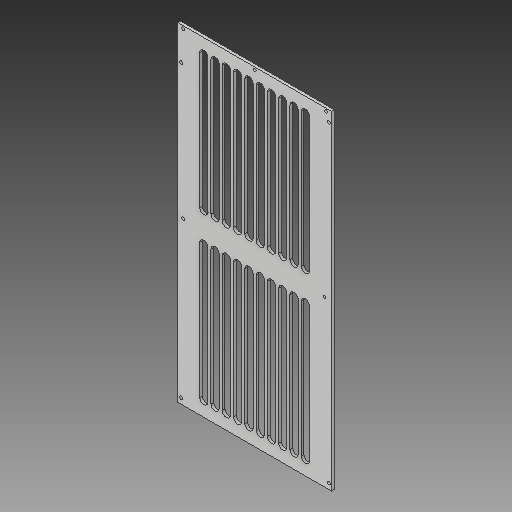
# Autodesk Inventor part: GlyphPlateUnderside
Saved by Autodesk Inventor 2019 (Build 230136000, 136)
## iProperties
Created: 2018-01-27
Part Number: GlyphPlateUnderside
Material: Generic
Document SubType Name: Modeling
Designer: User
Density: 1 g/cm^3
Appearance: Default
Author: User
Autodesk Inventor part; units mm, degrees
ref_plane "YZ Plane" through (0, 0, 0) normal (1, 0, 0) x (0, 1, 0)
ref_plane "XZ Plane" through (0, 0, 0) normal (0, 1, 0) x (-1, 0, 0)
ref_plane "XY Plane" through (0, 0, 0) normal (0, 0, 1) x (1, 0, 0)
sketch "Sketch1" plane through (0, 0, 0) normal (0, 0, 1) x (1, 0, 0)
  line L0 (0, 0) -> (178.2064, 0)
  line L1 (178.2064, 0) -> (178.2064, 381)
  line L2 (178.2064, 381) -> (0, 381)
  line L3 (0, 381) -> (0, 0)
  dimension "d0" = 178.2064
  dimension "d1" = 381
  constraints: 8 end point, 2 parallel, 1 horizontal, 1 perpendicular
  measures "d0" distance of L2.end L1.end
  measures "d1" distance of L1.end L0.end
extrude "Extrusion1" add sketch "Sketch1" along normal blind 3.175
sketch "Sketch2" plane through (0, 0, 3.175) normal (0, 0, 1) x (1, 0, 0)
  line L0 (0, 0) -> (178.2064, 0) projected
  line L1 (0, 0) -> (4.0386, 0)
  line L2 (4.0386, 0) -> (4.0386, 6.35)
  line L3 (0, 381) -> (0, 0) projected
  line L4 (0, 381) -> (4.0386, 381)
  line L5 (178.2064, 381) -> (0, 381) projected
  line L6 (4.0386, 381) -> (4.0386, 342.9)
  line L7 (4.0386, 381) -> (42.1386, 381) construction
  line L8 (0, 381) -> (0, 377.825)
  line L9 (0, 377.825) -> (6.35, 377.825)
  line L10 (178.2064, 0) -> (178.2064, 381) projected
  line L11 (178.2064, 0) -> (175.0314, 0)
  line L12 (175.0314, 0) -> (175.0314, 6.35)
  line L13 (178.2064, 377.825) -> (171.8564, 377.825)
  point P0 (175.0314, 368.3)
  dimension "d4" = 4.0386
  dimension "d5" = 6.35
  dimension "d6" = 38.1
  dimension "d7" = 90
  dimension "d8" = 3.175
  dimension "d9" = 6.35
  dimension "d10" = 3.175
  dimension "d11" = 6.35
  dimension "d19" = 4.0386
  dimension "d21" = 3.175
  dimension "d22" = 12.7
  dimension "d23" = 3.175
  constraints: 20 end point, 5 coincident, 5 perpendicular, 5 point on line, 1 horizontal, 1 vertical
  measures "d4" distance of L0.start L1.end
  measures "d5" distance of L1.end L2.end
  measures "d6" distance of L4.end L6.end
  measures "d7" angle of L6 L7
  measures "d8" distance of L3.start L8.end
  measures "d9" distance of L8.end L9.end
  measures "d10" distance of L0.end L11.end
  measures "d11" distance of L13.start L13.end
  measures "d19" distance between parallel lines of L3 L6
  measures "d21" distance from line of L10 point (175.031, 368.3)
  measures "d22" distance from line of point (175.031, 368.3) L5
  measures "d23" distance from line of L5 L13.end
hole "Hole1" at (4.0386, 6.35, 3.175) at (4.0386, 342.9, 3.175) at (6.35, 377.825, 3.175) at (175.0314, 6.35, 3.175) at (175.0314, 368.3, 3.175) at (171.8564, 377.825, 3.175) direction (0, 0, -1) diameter 3.556 depth 25.4 tip angle 118
sketch "Sketch3" plane through (0, 0, 3.175) normal (0, 0, 1) x (1, 0, 0)
  line L0 (30.1625, 12.7) -> (30.1625, 177.8) construction
  line L1 (34.925, 17.4625) -> (34.925, 173.0375)
  line L2 (25.4, 173.0375) -> (25.4, 17.4625)
  arc A0 (25.4, 17.4625) -> (34.925, 17.4625) centre (30.1625, 17.4625) ccw
  arc A1 (34.925, 173.0375) -> (25.4, 173.0375) centre (30.1625, 173.0375) ccw
  line L3 (0, 381) -> (0, 0) projected
  line L4 (178.2064, 0) -> (178.2064, 381) projected
  line L5 (0, 0) -> (178.2064, 0) projected
  line L6 (43.2435, 12.7) -> (43.2435, 177.8) construction
  line L7 (48.006, 17.4625) -> (48.006, 173.0375)
  line L8 (38.481, 173.0375) -> (38.481, 17.4625)
  arc A2 (38.481, 17.4625) -> (48.006, 17.4625) centre (43.2435, 17.4625) ccw
  arc A3 (48.006, 173.0375) -> (38.481, 173.0375) centre (43.2435, 173.0375) ccw
  line L9 (56.3245, 12.7) -> (56.3245, 177.8) construction
  line L10 (61.087, 17.4625) -> (61.087, 173.0375)
  line L11 (51.562, 173.0375) -> (51.562, 17.4625)
  arc A4 (51.562, 17.4625) -> (61.087, 17.4625) centre (56.3245, 17.4625) ccw
  arc A5 (61.087, 173.0375) -> (51.562, 173.0375) centre (56.3245, 173.0375) ccw
  line L12 (69.4055, 12.7) -> (69.4055, 177.8) construction
  line L13 (74.168, 17.4625) -> (74.168, 173.0375)
  line L14 (64.643, 173.0375) -> (64.643, 17.4625)
  arc A6 (64.643, 17.4625) -> (74.168, 17.4625) centre (69.4055, 17.4625) ccw
  arc A7 (74.168, 173.0375) -> (64.643, 173.0375) centre (69.4055, 173.0375) ccw
  line L15 (82.4865, 12.7) -> (82.4865, 177.8) construction
  line L16 (87.249, 17.4625) -> (87.249, 173.0375)
  line L17 (77.724, 173.0375) -> (77.724, 17.4625)
  arc A8 (77.724, 17.4625) -> (87.249, 17.4625) centre (82.4865, 17.4625) ccw
  arc A9 (87.249, 173.0375) -> (77.724, 173.0375) centre (82.4865, 173.0375) ccw
  line L18 (95.5675, 12.7) -> (95.5675, 177.8) construction
  line L19 (100.33, 17.4625) -> (100.33, 173.0375)
  line L20 (90.805, 173.0375) -> (90.805, 17.4625)
  arc A10 (90.805, 17.4625) -> (100.33, 17.4625) centre (95.5675, 17.4625) ccw
  arc A11 (100.33, 173.0375) -> (90.805, 173.0375) centre (95.5675, 173.0375) ccw
  line L21 (108.6485, 12.7) -> (108.6485, 177.8) construction
  line L22 (113.411, 17.4625) -> (113.411, 173.0375)
  line L23 (103.886, 173.0375) -> (103.886, 17.4625)
  arc A12 (103.886, 17.4625) -> (113.411, 17.4625) centre (108.6485, 17.4625) ccw
  arc A13 (113.411, 173.0375) -> (103.886, 173.0375) centre (108.6485, 173.0375) ccw
  line L24 (121.7295, 12.7) -> (121.7295, 177.8) construction
  line L25 (126.492, 17.4625) -> (126.492, 173.0375)
  line L26 (116.967, 173.0375) -> (116.967, 17.4625)
  arc A14 (116.967, 17.4625) -> (126.492, 17.4625) centre (121.7295, 17.4625) ccw
  arc A15 (126.492, 173.0375) -> (116.967, 173.0375) centre (121.7295, 173.0375) ccw
  line L27 (160.7328, 14.2764) -> (160.7328, 166.6986) construction
  line L28 (134.8105, 12.7) -> (134.8105, 177.8) construction
  line L29 (139.573, 17.4625) -> (139.573, 173.0375)
  line L30 (130.048, 173.0375) -> (130.048, 17.4625)
  arc A16 (130.048, 17.4625) -> (139.573, 17.4625) centre (134.8105, 17.4625) ccw
  arc A17 (139.573, 173.0375) -> (130.048, 173.0375) centre (134.8105, 173.0375) ccw
  line L31 (178.2064, 0) -> (178.2064, 381) projected
  line L32 (30.1625, 368.3) -> (30.1625, 203.2) construction
  line L33 (34.925, 363.5375) -> (34.925, 207.9625)
  line L34 (25.4, 207.9625) -> (25.4, 363.5375)
  arc A18 (34.925, 363.5375) -> (25.4, 363.5375) centre (30.1625, 363.5375) ccw
  arc A19 (25.4, 207.9625) -> (34.925, 207.9625) centre (30.1625, 207.9625) ccw
  arc A20 (38.481, 207.9625) -> (48.006, 207.9625) centre (43.2435, 207.9625) ccw
  line L35 (48.006, 363.5375) -> (48.006, 207.9625)
  line L36 (38.481, 207.9625) -> (38.481, 363.5375)
  line L37 (43.2435, 368.3) -> (43.2435, 203.2) construction
  arc A21 (48.006, 363.5375) -> (38.481, 363.5375) centre (43.2435, 363.5375) ccw
  arc A22 (51.562, 207.9625) -> (61.087, 207.9625) centre (56.3245, 207.9625) ccw
  line L38 (61.087, 363.5375) -> (61.087, 207.9625)
  line L39 (51.562, 207.9625) -> (51.562, 363.5375)
  line L40 (56.3245, 368.3) -> (56.3245, 203.2) construction
  arc A23 (61.087, 363.5375) -> (51.562, 363.5375) centre (56.3245, 363.5375) ccw
  arc A24 (64.643, 207.9625) -> (74.168, 207.9625) centre (69.4055, 207.9625) ccw
  line L41 (74.168, 363.5375) -> (74.168, 207.9625)
  line L42 (64.643, 207.9625) -> (64.643, 363.5375)
  line L43 (69.4055, 368.3) -> (69.4055, 203.2) construction
  arc A25 (74.168, 363.5375) -> (64.643, 363.5375) centre (69.4055, 363.5375) ccw
  arc A26 (77.724, 207.9625) -> (87.249, 207.9625) centre (82.4865, 207.9625) ccw
  line L44 (87.249, 363.5375) -> (87.249, 207.9625)
  line L45 (77.724, 207.9625) -> (77.724, 363.5375)
  line L46 (82.4865, 368.3) -> (82.4865, 203.2) construction
  arc A27 (87.249, 363.5375) -> (77.724, 363.5375) centre (82.4865, 363.5375) ccw
  arc A28 (90.805, 207.9625) -> (100.33, 207.9625) centre (95.5675, 207.9625) ccw
  line L47 (100.33, 363.5375) -> (100.33, 207.9625)
  line L48 (90.805, 207.9625) -> (90.805, 363.5375)
  line L49 (95.5675, 368.3) -> (95.5675, 203.2) construction
  arc A29 (100.33, 363.5375) -> (90.805, 363.5375) centre (95.5675, 363.5375) ccw
  arc A30 (103.886, 207.9625) -> (113.411, 207.9625) centre (108.6485, 207.9625) ccw
  line L50 (113.411, 363.5375) -> (113.411, 207.9625)
  line L51 (103.886, 207.9625) -> (103.886, 363.5375)
  line L52 (108.6485, 368.3) -> (108.6485, 203.2) construction
  arc A31 (113.411, 363.5375) -> (103.886, 363.5375) centre (108.6485, 363.5375) ccw
  arc A32 (116.967, 207.9625) -> (126.492, 207.9625) centre (121.7295, 207.9625) ccw
  line L53 (126.492, 363.5375) -> (126.492, 207.9625)
  line L54 (116.967, 207.9625) -> (116.967, 363.5375)
  line L55 (121.7295, 368.3) -> (121.7295, 203.2) construction
  arc A33 (126.492, 363.5375) -> (116.967, 363.5375) centre (121.7295, 363.5375) ccw
  arc A34 (130.048, 207.9625) -> (139.573, 207.9625) centre (134.8105, 207.9625) ccw
  line L56 (139.573, 363.5375) -> (139.573, 207.9625)
  line L57 (130.048, 207.9625) -> (130.048, 363.5375)
  line L58 (134.8105, 368.3) -> (134.8105, 203.2) construction
  arc A35 (139.573, 363.5375) -> (130.048, 363.5375) centre (134.8105, 363.5375) ccw
  line L59 (147.8915, 12.7) -> (147.8915, 177.8) construction
  line L60 (152.654, 17.4625) -> (152.654, 173.0375)
  line L61 (143.129, 173.0375) -> (143.129, 17.4625)
  arc A36 (143.129, 17.4625) -> (152.654, 17.4625) centre (147.8915, 17.4625) ccw
  arc A37 (152.654, 173.0375) -> (143.129, 173.0375) centre (147.8915, 173.0375) ccw
  arc A38 (143.129, 207.9625) -> (152.654, 207.9625) centre (147.8915, 207.9625) ccw
  line L62 (152.654, 363.5375) -> (152.654, 207.9625)
  line L63 (143.129, 207.9625) -> (143.129, 363.5375)
  line L64 (147.8915, 368.3) -> (147.8915, 203.2) construction
  arc A39 (152.654, 363.5375) -> (143.129, 363.5375) centre (147.8915, 363.5375) ccw
  point P0 (30.1625, 95.25)
  point P1 (43.2435, 95.25)
  point P2 (56.3245, 95.25)
  point P3 (69.4055, 95.25)
  point P4 (82.4865, 95.25)
  point P5 (95.5675, 95.25)
  point P6 (108.6485, 95.25)
  point P7 (121.7295, 95.25)
  point P8 (144.4212, 90.4875)
  point P9 (134.8105, 95.25)
  point P10 (36.7792, 292.1)
  point P11 (49.8602, 292.1)
  point P12 (62.9412, 292.1)
  point P13 (76.0222, 292.1)
  point P14 (89.1032, 292.1)
  point P15 (102.1842, 292.1)
  point P16 (115.2652, 292.1)
  point P17 (128.3462, 292.1)
  point P18 (141.4272, 292.1)
  point P19 (147.8915, 95.25)
  point P20 (154.5082, 292.1)
  dimension "d24" = 9.525
  dimension "d34" = 12.7
  dimension "d39" = 381
  dimension "d41" = 165.1
  dimension "d46" = 13.081
  dimension "d55" = 13.081
  dimension "d63" = 165.1
  dimension "d64" = 25.4
  dimension "d65" = 25.4
  constraints: 164 end point, 120 point on circle, 40 centre point, 40 point on line, 4 tangent, 2 horizontal, 1 midpoint, 1 parallel, 1 vertical, 252 other
  measures "d24" diameter of A1
  measures "d34" distance from line of L5 L0.start
  measures "d39" distance of L4.start L4.end
  measures "d41" distance of L0.start L0.end
  measures "d46" distance of L1.start L7.start
  measures "d55" distance of L32.end L37.end
  measures "d63" distance of L32.end L32.start
  measures "d64" distance between parallel lines of L3 L2
  measures "d65" distance between parallel lines of L3 L34
extrude "Extrusion2" cut sketch "Sketch3" against normal through all
sketch "Sketch4" plane through (0, 0, 3.175) normal (0, 0, 1) x (1, 0, 0)
  circle A0 centre (6.35, 377.825) radius 1.778 projected
  circle A1 centre (6.35, 187.325) radius 1.778
  circle A2 centre (89.1032, 377.825) radius 1.778
  line L0 (0, 0) -> (178.2064, 0) projected
  line L1 (0, 381) -> (0, 0) projected
  circle A3 centre (170.0784, 190.5) radius 1.778
  dimension "d66" = 3.556
  dimension "d68" = 3.556
  dimension "d72" = 187.325
  dimension "d74" = 82.7532
  dimension "d75" = 3.556
  constraints: 3 centre point
  measures "d66" diameter of A1
  measures "d68" diameter of A2
  measures "d72" distance from line of L0 A1.centre
  measures "d74" distance of A2.centre A0.centre
  measures "d75" diameter of A3
extrude "Extrusion3" cut sketch "Sketch4" against normal blind 3.556
equation "\"d69\" = d75"
body "Solid1"
